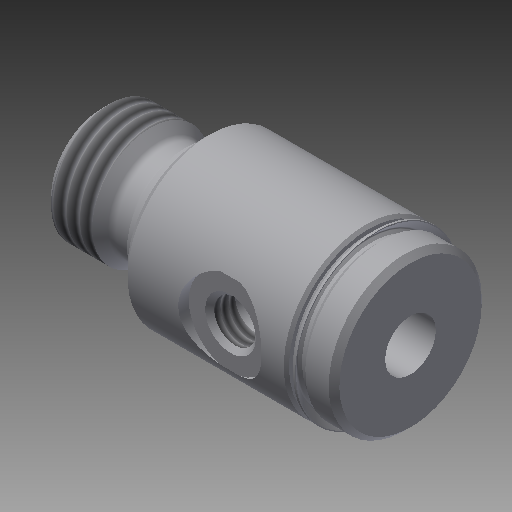
# Autodesk Inventor part: 02R010-0_rod_guide
Saved by Autodesk Inventor 2018 (Build 220112000, 112)
## iProperties
Category: PARTsolutions
Company: BIMBA
Created: 2019-01-18
Part Number: 02R010-0_rod_guide
Material: Generic
Catalog Web Link: www.cadenas.de
Description: Rod Guide-Original Line - Standard Air Cylinders
Vendor: BIMBA
Document SubType Name: Modeling
Designer: psadmin
Manufacturer: BIMBA
Mass: 3.85898 g
Surface Area: 21.9957 cm^2
Volume: 3.85898 cm^3
Density: 1 g/cm^3
Appearance: PSOLRGB-211-211-211
PSOL_IDENT_0: {$CADENAS_DATA\23d-libs\bimba\bimba\bimba_imperial\bimba_full_line\original_line_cylinders\standard_
PSOL_IDENT_1: air_cylinders\rod_guide.prj},251 {VTYP=3D},{NB=02R010-0_rod_guide},{LINA=02R010-0_rod_guide},{NN=Rod
PSOL_IDENT_2: Guide},{DATE=21.03.2018 14:31:21},{GEOMDATE=09.11.2017 12:44:00},{VERSION=},{LINEID=30},{WBVAR=MNT,
PSOL_IDENT_3: ACTING,NR,K,Q,T1,T2,T3,T4,MB,TRIM,CUSH,RODTRANS},{WBNUMERIC=MB,TRIM,CUSH,RODTRANS}  {NB=02R010-0_rod
PSOL_IDENT_4: _guide},{LINA=02R010-0_rod_guide},{KT=DUMMY},{PN=02R010},{BORE=0.56250000},{BOREPN=02},{MNT=},{MNTAL
PSOL_IDENT_5: G='' , 'Front Nose'},{ACTING=R},{ACTINGALG= '' , 'Single Acting' , 'R' , 'Reverse/Double Acting' },{
PSOL_IDENT_6: NR=},{NRALG= '' , 'N/A' },{K=},{Q=},{QALG= '' , 'Without Side Ported Rear Head' , 'Q' , 'With Side P
PSOL_IDENT_7: orted Rear Head' },{T1=},{T2=},{T3=},{T4=},{MB=1},{A1=1.1560},{A1N=1.0310},{A1P=1.1560},{A1B=0.0000}
PSOL_IDENT_8: ,{A2=0.3750},{A2N=0.3750},{A2P=0.3750},{A3=0.6250},{A3N=0.1250},{A3P=0.6250},{A4=0.1570},{A4N=0.5310
PSOL_IDENT_9: },{A4P=0.1570},{A5=0.0250},{A6=0.0000},{A6N=0.2810},{A6P=0.0000},{A7=0.5000},{A7N=0.6560},{A7P=0.500
PSOL_IDENT_10: 0},{A8=0.0200},{A8N=0.0200},{A8NR=0.0200},{D1=0.6150},{D1N=0.6150},{D1P=0.6150},{D1B=0.0000},{D2=0.5
PSOL_IDENT_11: 725},{D3=0.0000},{D3N=0.4000},{D3P=0.0000},{D4=0.3440},{D4N=0.2220},{D4P=0.3440},{D4NR=0.3440},{D5=0
PSOL_IDENT_12: .1900},{D5N=0.1900},{D5NR=0.1900},{C1=0.030},{C2=0.0200},{C2N=0.0300},{C2P=0.0200},{C3=0.0100},{C3N=
PSOL_IDENT_13: 0.0100},{C3P=0.0100},{C4=0.0300},{C4N=0.0300},{C4P=0.0300},{NDM=0.4375},{NDMN=0.4375},{NDMP=0.4375},
PSOL_IDENT_14: {TAB=UNF},{D6=0.4355},{D6N=0.4355},{D6P=0.4355},{A9=0.0620},{A9N=0.0620},{A9P=0.0620},{D7=0.3600},{D
PSOL_IDENT_15: 7N=0.3600},{D7P=0.3600},{A10=0.0775},{A10N=0.0775},{A10P=0.0775},{R1=0.0315},{R1N=0.0315},{R1P=0.031
PSOL_IDENT_16: 5},{D8=0.0000},{D9=0.0000},{D10=0.0000},{A11=0.0000},{A12=0.0000},{A13=0.0000},{A14=0.4060},{A14N=0.
PSOL_IDENT_17: 4060},{A14B=0.0000},{D11=0.0000},{D11N=0.0000},{NDM2=0.1900},{NDM2N=0.1900},{NDM2DP=0.0000},{THREAD=
PSOL_IDENT_18: 0},{HEX=0.1920},{HEXN=0.1920},{S1=0.0000},{B1=0.0000},{B2=0.0000},{B22=0.0000},{DB=0.0000},{B3=0.000
PSOL_IDENT_19: 0},{B4=0.0000},{X1=0.0000},{X2=0.0000},{NDM3=0.0000},{NDM4=0.0000},{NDM4DP=0.0000},{DD=0.0000},{CB=0
PSOL_IDENT_20: .0000},{CBDP=0.0000},{PORT=1},{XT=0.0000},{XTX=0.0000},{XT1=0.0000},{XT2=0.0000},{NDMH=0.0000},{OD=0
PSOL_IDENT_21: .6150},{ID=0.5725},{G=0.0000},{PNUT=0.3750},{TRIM=0},{C11=0.0000},{C22=0.0000},{C33=0.0000},{C44=0.0
PSOL_IDENT_22: 000},{C55=0.0000},{CD1=0.0000},{CD2=0.0000},{CD3=0.0000},{CNDM3=0.0000},{CTAB3=0.0000},{CUSH=0},{XX=
PSOL_IDENT_23: 0.00000},{LCD=0.0000},{RODTRANS=0.00000}
NN: Rod Guide
NT: Original Line - Standard Air Cylinders
NB: 02R010-0_rod_guide
NBSYN: $PN.-$RODTRANS._rod_guide
LINA: 02R010-0_rod_guide
BORE: 0
BOREPN: 02
MNT: Front Nose
MNTALG: '' , 'Front Nose'
ACTING: Reverse/Double Acting
NR: N/A
K: Standard
Q: Without Side Ported Rear Head
T1: without T1
T2: without T2
T3: without T3
T4: without T4
MB: 1
A1N: 1.031
A1P: 1.156
A1B: 0
A2N: 0.375
A2P: 0.375
A3N: 0.125
A3P: 0.625
A4N: 0.531
A4P: 0.157
A5: 0.025
A6N: 0.281
A6P: 0
A7N: 0.656
A7P: 0.5
A8N: 0.02
A8NR: 0.02
D1N: 0.615
D1P: 0.615
D1B: 0
D2: 0.5725
D3N: 0.4
D3P: 0
D4N: 0.222
D4P: 0.344
D4NR: 0.344
D5N: 0.19
D5NR: 0.19
C1: 0.03
C2N: 0.03
C2P: 0.02
C3N: 0.01
C3P: 0.01
C4N: 0.03
C4P: 0.03
NDMN: 0.4375
NDMP: 0.4375
TAB: UNF
D6N: 0.4355
D6P: 0.4355
A9N: 0.062
A9P: 0.062
D7N: 0.36
D7P: 0.36
A10N: 0.0775
A10P: 0.0775
R1N: 0.0315
R1P: 0.0315
D8: 0
D9: 0
D10: 0
A11: 0
A12: 0
A13: 0
A14N: 0.406
A14B: 0
D11N: 0
NDM2N: 0.19
NDM2DP: 0
HEXN: 0.192
S1: 0
B1: 0
B2: 0
B22: 0
DB: 0
B3: 0
B4: 0
X1: 0
X2: 0
NDM3: 0
NDM4: 0
NDM4DP: 0
DD: 0
CB: 0
CBDP: 0
XTX: 0
XT1: 0
XT2: 0
NDMH: 0
TRIM: 0
C11: 0
C22: 0
C33: 0
C44: 0
C55: 0
CD1: 0
CD2: 0
CD3: 0
CNDM3: 0
CTAB3: 0.0000
CUSH: 0
LCD: 0
RODTRANS: 0
SUPPLIER: BIMBA
ARTICLENO: 02R010-0_rod_guide
BOMINFO: 02R010-0_rod_guide
CREATOR: CADENAS GmbH
Title: 02R010-0_rod_guide
Author: Cadenas PARTsolutions
Comments: Original Line - Standard Air Cylinders
Autodesk Inventor part; units mm, degrees
sketch "Sketch_2" plane through (0, 0, 0) normal (0, 0, 1) x (1, 0, 0)
  line L0 (9.525, 0) -> (0, 0)
  line L1 (0, 0) -> (0, 4.8006)
  line L2 (0, 4.8006) -> (0.7557, 5.5563)
  line L3 (0.7557, 5.5563) -> (4.6603, 5.5563)
  line L4 (4.6603, 5.5563) -> (5.4181, 4.8042)
  arc A0 (5.4181, 4.8042) -> (5.9817, 4.572) centre (5.9817, 5.3721) ccw
  line L5 (5.9817, 4.572) -> (7.1501, 4.572)
  arc A1 (7.1501, 4.572) -> (7.9502, 5.3721) centre (7.1501, 5.3721) ccw
  line L6 (7.9502, 5.3721) -> (7.9502, 5.5309)
  line L7 (7.9502, 5.5309) -> (9.525, 5.5309)
  line L8 (9.525, 5.5309) -> (9.525, 0)
  line L9 (9.525, 0) -> (0, 0)
  constraints: 20 end point, 4 point on circle, 2 centre point
revolve "Revolution1" add sketch "Sketch_2" angle 360 about axis through (9.525, 0, 0) along (1, 0, 0)
thread "Thread1" size "7/16-20 UNF" class "2A" standard "ANSI Unified Screw Threads" full length
sketch "Sketch_3" plane through (0, 0, 0) normal (0, 0, 1) x (1, 0, 0)
  line L0 (29.3624, 0) -> (9.525, 0)
  line L1 (9.525, 0) -> (9.525, 7.0485)
  line L2 (9.525, 7.0485) -> (10.287, 7.8105)
  line L3 (10.287, 7.8105) -> (25.1206, 7.8105)
  line L4 (25.1206, 7.8105) -> (25.3746, 7.5565)
  line L5 (25.3746, 7.5565) -> (25.3746, 6.6357)
  line L6 (25.3746, 6.6357) -> (26.0096, 6.6357)
  line L7 (26.0096, 6.6357) -> (26.6446, 7.2708)
  line L8 (26.6446, 7.2708) -> (28.8544, 7.2708)
  line L9 (28.8544, 7.2708) -> (29.3624, 6.7627)
  line L10 (29.3624, 6.7627) -> (29.3624, 0)
  line L11 (29.3624, 0) -> (9.525, 0)
  constraints: 24 end point
revolve "Revolution2" add sketch "Sketch_3" angle 360 about axis through (29.3624, 0, 0) along (1, 0, 0)
sketch "Sketch3" plane through (0, 0, 0) normal (-1, 0, 0) x (0, 0, 1)
  point P0 (0, 0)
hole "Hole1" at (0, 0, 0) direction (1, 0, 0) diameter 4.826 depth 29.3624 countersink diameter 5.842 countersink angle 90
sketch "Sketch_12" plane through (0, 0, 0) normal (0, 1, 0) x (-1, 0, 0)
  line L0 (-19.05, 7.8105) -> (-19.05, -1.016)
  line L1 (-19.05, -1.016) -> (-21.0337, -1.016)
  line L2 (-21.0337, -1.016) -> (-21.0337, 6.3652)
  line L3 (-21.0337, 6.3652) -> (-21.463, 6.7945)
  line L4 (-21.463, 6.7945) -> (-23.0124, 6.7945)
  line L5 (-23.0124, 6.7945) -> (-23.0124, 7.8105)
  line L6 (-23.0124, 7.8105) -> (-19.05, 7.8105)
  line L7 (-19.05, 7.8105) -> (-19.05, -1.016)
  constraints: 16 end point
revolve "Revolution3" cut sketch "Sketch_12" angle 360 about axis through (19.05, 0, 7.8105) along (0, 0, 1)
thread "Thread2" size "10-32 UNF" class "2B" standard "ANSI Unified Screw Threads" length 1.9964
sketch "Sketch_47" plane through (0, 0, 0) normal (0, 0, 1) x (1, 0, 0)
  line L0 (26.0096, 0) -> (25.3746, 0)
  line L1 (25.3746, 7.1861) -> (25.3746, 6.3818)
  line L2 (25.3746, 6.3818) -> (26.0096, 6.3818)
  line L3 (26.0096, 6.3818) -> (26.0096, 6.6357)
  line L4 (26.0096, 6.6357) -> (25.6921, 6.6357)
  line L5 (25.6921, 6.6357) -> (25.4916, 6.8362)
  arc A0 (25.4916, 7.0158) -> (25.4916, 6.8362) centre (25.5814, 6.926) ccw
  line L6 (25.4916, 7.0158) -> (26.2022, 7.7263)
  line L7 (26.2022, 7.7263) -> (26.2022, 7.8105)
  line L8 (26.2022, 7.8105) -> (25.999, 7.8105)
  line L9 (25.999, 7.8105) -> (25.3746, 7.1861)
  constraints: 20 end point, 2 point on circle, 1 centre point
revolve "Revolution4" add sketch "Sketch_47" angle 360 about axis through (26.0096, 0, 0) along (1, 0, 0)
ref_plane "dp1_XY" through (9.525, 5.5309, 0) normal (0, 0, 1) x (1, 0, 0)
ref_plane "dp1_YZ" through (9.525, 5.5309, 0) normal (1, 0, 0) x (0, 1, 0)
ref_plane "dp1_ZX" through (9.525, 5.5309, 0) normal (0, 1, 0) x (0, 0, 1)
ref_plane "dp2_XY" through (9.525, -5.5309, 0) normal (0, 0, 1) x (1, 0, 0)
ref_plane "dp2_YZ" through (9.525, -5.5309, 0) normal (1, 0, 0) x (0, 1, 0)
ref_plane "dp2_ZX" through (9.525, -5.5309, 0) normal (0, 1, 0) x (0, 0, 1)
ref_plane "hh_XY" through (0, 5.5563, 0) normal (0, 0, 1) x (1, 0, 0)
ref_plane "hh_YZ" through (0, 5.5563, 0) normal (1, 0, 0) x (0, 1, 0)
ref_plane "hh_ZX" through (0, 5.5563, 0) normal (0, 1, 0) x (0, 0, 1)
ref_plane "port_XY" through (19.05, 0, 0) normal (0, 0, 1) x (1, 0, 0)
ref_plane "port_YZ" through (19.05, 0, 0) normal (1, 0, 0) x (0, 1, 0)
ref_plane "port_ZX" through (19.05, 0, 0) normal (0, 1, 0) x (0, 0, 1)
ref_plane "rod_guide_XY" through (0, 0, 0) normal (1, 0, 0) x (0, 0, -1)
ref_plane "rod_guide_YZ" through (0, 0, 0) normal (0, 0, -1) x (0, 1, 0)
ref_plane "rod_guide_ZX" through (0, 0, 0) normal (0, 1, 0) x (1, 0, 0)
ref_plane "s1_XY" through (7.9502, 0, 0) normal (0, 0, 1) x (1, 0, 0)
ref_plane "s1_YZ" through (7.9502, 0, 0) normal (1, 0, 0) x (0, 1, 0)
ref_plane "s1_ZX" through (7.9502, 0, 0) normal (0, 1, 0) x (0, 0, 1)
ref_plane "s2_XY" through (9.525, 0, 0) normal (0, 0, 1) x (1, 0, 0)
ref_plane "s2_YZ" through (9.525, 0, 0) normal (1, 0, 0) x (0, 1, 0)
ref_plane "s2_ZX" through (9.525, 0, 0) normal (0, 1, 0) x (0, 0, 1)
ref_plane "t1_XY" through (9.525, 0, 0) normal (1, 0, 0) x (0, 0, -1)
ref_plane "t1_YZ" through (9.525, 0, 0) normal (0, 0, -1) x (0, 1, 0)
ref_plane "t1_ZX" through (9.525, 0, 0) normal (0, 1, 0) x (1, 0, 0)
ref_plane "t111_XY" through (9.525, 0, 0) normal (1, 0, 0) x (0, 0, -1)
ref_plane "t111_YZ" through (9.525, 0, 0) normal (0, 0, -1) x (0, 1, 0)
ref_plane "t111_ZX" through (9.525, 0, 0) normal (0, 1, 0) x (1, 0, 0)
ref_plane "to_foot_bracket_XY" through (9.525, 0, 0) normal (1, 0, 0) x (0, 0, -1)
ref_plane "to_foot_bracket_YZ" through (9.525, 0, 0) normal (0, 0, -1) x (0, 1, 0)
ref_plane "to_foot_bracket_ZX" through (9.525, 0, 0) normal (0, 1, 0) x (1, 0, 0)
ref_plane "to_nut_XY" through (9.525, 0, 0) normal (1, 0, 0) x (0, 0, -1)
ref_plane "to_nut_YZ" through (9.525, 0, 0) normal (0, 0, -1) x (0, 1, 0)
ref_plane "to_nut_ZX" through (9.525, 0, 0) normal (0, 1, 0) x (1, 0, 0)
ref_plane "to_rod_XY" through (0, 0, 0) normal (1, 0, 0) x (0, 0, -1)
ref_plane "to_rod_YZ" through (0, 0, 0) normal (0, 0, -1) x (0, 1, 0)
ref_plane "to_rod_ZX" through (0, 0, 0) normal (0, 1, 0) x (1, 0, 0)
ref_plane "to_screw_XY" through (19.05, 0, 0) normal (0, 1, 0) x (1, 0, 0)
ref_plane "to_screw_YZ" through (19.05, 0, 0) normal (1, 0, 0) x (0, 0, -1)
ref_plane "to_screw_ZX" through (19.05, 0, 0) normal (0, 0, -1) x (0, 1, 0)
ref_plane "to_trunnion_brackets_XY" through (0, 0, 0) normal (0, 1, 0) x (1, 0, 0)
ref_plane "to_trunnion_brackets_YZ" through (0, 0, 0) normal (1, 0, 0) x (0, 0, -1)
ref_plane "to_trunnion_brackets_ZX" through (0, 0, 0) normal (0, 0, -1) x (0, 1, 0)
ref_plane "to_trunnion_brackets1_XY" through (0, 0, 0) normal (0, 1, 0) x (1, 0, 0)
ref_plane "to_trunnion_brackets1_YZ" through (0, 0, 0) normal (1, 0, 0) x (0, 0, -1)
ref_plane "to_trunnion_brackets1_ZX" through (0, 0, 0) normal (0, 0, -1) x (0, 1, 0)
ref_plane "to_trunnion_brackets2_XY" through (0, 0, 0) normal (0, 1, 0) x (1, 0, 0)
ref_plane "to_trunnion_brackets2_YZ" through (0, 0, 0) normal (1, 0, 0) x (0, 0, -1)
ref_plane "to_trunnion_brackets2_ZX" through (0, 0, 0) normal (0, 0, -1) x (0, 1, 0)
ref_plane "to_tube_XY" through (26.0096, 0, 0) normal (1, 0, 0) x (0, 0, -1)
ref_plane "to_tube_YZ" through (26.0096, 0, 0) normal (0, 0, -1) x (0, 1, 0)
ref_plane "to_tube_ZX" through (26.0096, 0, 0) normal (0, 1, 0) x (1, 0, 0)
body "Solid1"
